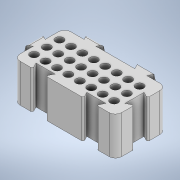
# Autodesk Inventor part: 4x11mmFlatBottom
Saved by Autodesk Inventor 2022.2 (Build 262287010, 287A)
## iProperties
Part Number: 4x11mmFlatBottom
Material: Generic
Document SubType Name: Modeling
Designer: yiunf
Appearance: Default
Author: yiunf
## iProperties of the stored document 4x8mm_3DPrint.ipt
Part Number: 4x8mm_3DPrint
Material: Generic
Document SubType Name: Modeling
Designer: yiunf
Appearance: Default
Author: yiunf
Autodesk Inventor part; units mm, degrees
ref_plane "YZ Plane" through (0, 0, 0) normal (1, 0, 0) x (0, 1, 0)
ref_plane "XZ Plane" through (0, 0, 0) normal (0, 1, 0) x (-1, 0, 0)
ref_plane "XY Plane" through (0, 0, 0) normal (0, 0, 1) x (1, 0, 0)
sketch "Sketch1" plane through (0, 0, 0) normal (0, 1, 0) x (-1, 0, 0)
  line L0 (-40, -20) -> (40, -20)
  line L1 (40, -20) -> (40, 20)
  line L2 (40, 20) -> (-40, 20)
  line L3 (-40, 20) -> (-40, -20)
  line L4 (-40, -20) -> (40, 20) construction
  line L5 (40, -20) -> (-40, 20) construction
  line L6 (40, 0) -> (45, 0)
  line L7 (45, 0) -> (45, 7.5)
  line L8 (40, 0) -> (40, 5)
  line L9 (40, 5) -> (45, 7.5)
  line L10 (45, 0) -> (45, -7.5)
  line L11 (40, 0) -> (40, -5)
  line L12 (40, -5) -> (45, -7.5)
  line L13 (0, -20) -> (5, -20)
  line L14 (0, -20) -> (-5, -20)
  line L15 (0, -20) -> (0, -25)
  line L16 (0, -25) -> (7.5, -25)
  line L17 (7.5, -25) -> (5, -20)
  line L18 (0, -25) -> (-7.5, -25)
  line L19 (-7.5, -25) -> (-5, -20)
  line L20 (-35, 0) -> (-35, -7.5)
  line L21 (-40, -5) -> (-35, -7.5)
  line L22 (-40, 0) -> (-35, 0)
  line L23 (-35, 0) -> (-35, 7.5)
  line L24 (-40, 5) -> (-35, 7.5)
  line L25 (-7.5, 15) -> (-5, 20)
  line L26 (0, 15) -> (-7.5, 15)
  line L27 (0, 20) -> (0, 15)
  line L28 (7.5, 15) -> (5, 20)
  line L29 (0, 15) -> (7.5, 15)
  line L30 (27.5, -25) -> (25, -20)
  line L31 (20, -25) -> (27.5, -25)
  line L32 (20, -25) -> (12.5, -25)
  line L33 (12.5, -25) -> (15, -20)
  line L34 (20, -20) -> (20, -25)
  line L35 (7.5, 15) -> (5, 20)
  line L36 (0, 15) -> (7.5, 15)
  line L37 (0, 15) -> (-7.5, 15)
  line L38 (-7.5, 15) -> (-5, 20)
  line L39 (0, 20) -> (0, 15)
  line L40 (27.5, 15) -> (25, 20)
  line L41 (20, 15) -> (27.5, 15)
  line L42 (20, 15) -> (12.5, 15)
  line L43 (12.5, 15) -> (15, 20)
  line L44 (20, 20) -> (20, 15)
  line L45 (-12.5, -25) -> (-15, -20)
  line L46 (-20, -25) -> (-12.5, -25)
  line L47 (-20, -20) -> (-20, -25)
  line L48 (-20, -25) -> (-27.5, -25)
  line L49 (-27.5, -25) -> (-25, -20)
  line L50 (7.5, 15) -> (5, 20)
  line L51 (0, 15) -> (7.5, 15)
  line L52 (0, 20) -> (0, 15)
  line L53 (0, 15) -> (-7.5, 15)
  line L54 (-7.5, 15) -> (-5, 20)
  line L55 (-12.5, 15) -> (-15, 20)
  line L56 (-20, 15) -> (-12.5, 15)
  line L57 (-20, 20) -> (-20, 15)
  line L58 (-20, 15) -> (-27.5, 15)
  line L59 (-27.5, 15) -> (-25, 20)
  line L60 (20, -24.75) -> (27.0955, -24.75)
  line L61 (27.0955, -24.75) -> (24.7764, -20.1118)
  line L62 (20, -24.75) -> (12.9045, -24.75)
  line L63 (12.9045, -24.75) -> (15.2236, -20.1118)
  line L64 (0, -24.5) -> (-6.691, -24.5)
  line L65 (-6.691, -24.5) -> (-4.691, -20.5)
  line L66 (-4.691, -20.5) -> (0, -20.5)
  line L67 (0, -24.75) -> (7.0955, -24.75)
  line L68 (7.0955, -24.75) -> (4.8455, -20.25)
  line L69 (4.8455, -20.25) -> (0, -20.25)
  line L70 (-20, -24.75) -> (-12.9045, -24.75)
  line L71 (-12.9045, -24.75) -> (-15.2236, -20.1118)
  line L72 (-20, -24.75) -> (-27.0955, -24.75)
  line L73 (-27.0955, -24.75) -> (-24.7764, -20.1118)
  line L74 (44.75, 0) -> (44.75, -7.0955)
  line L75 (44.75, -7.0955) -> (40.25, -4.8455)
  line L76 (40.25, -4.8455) -> (40.25, 0)
  line L77 (44.75, 0) -> (44.75, 7.0955)
  line L78 (44.75, 7.0955) -> (40.25, 4.8455)
  line L79 (40.25, 4.8455) -> (40.25, 0)
  line L80 (44.75, -7.0955) -> (40, -4.7205)
  line L81 (27.0955, -24.75) -> (24.7205, -20)
  line L82 (12.9045, -24.75) -> (15.2795, -20)
  line L83 (-12.9045, -24.75) -> (-15.2795, -20)
  line L84 (-27.0955, -24.75) -> (-24.7205, -20)
  line L85 (44.75, 7.0955) -> (40, 4.7205)
  line L86 (45, 0) -> (43.75, 0)
  line L87 (43.75, 0) -> (43.75, -6.875)
  line L88 (43.75, 0) -> (43.75, 6.875)
  line L89 (20, -25) -> (20, -23.75)
  line L90 (20, -23.75) -> (26.875, -23.75)
  line L91 (20, -23.75) -> (13.125, -23.75)
  line L92 (-20, -25) -> (-20, -23.75)
  line L93 (-20, -23.75) -> (-13.125, -23.75)
  line L94 (-20, -23.75) -> (-26.875, -23.75)
  point P0 (0, 0)
  point P1 (-40, -5)
  point P2 (24.7764, -20.1118)
  point P3 (40, -4.7205)
  point P4 (43.75, -6.5955)
  point P5 (43.75, 6.5955)
  point P6 (-26.5955, -23.75)
  point P7 (-13.4045, -23.75)
  point P8 (13.4045, -23.75)
  point P9 (26.5955, -23.75)
  dimension "d0" = 80
  dimension "d1" = 40
  dimension "d2" = 5
  dimension "d3" = 7.5
  dimension "d4" = 5
  dimension "d5" = 7.5
  dimension "d6" = 5
  dimension "d7" = 5
  dimension "d8" = 5
  dimension "d9" = 5
  dimension "d10" = 7.5
  dimension "d11" = 7.5
  dimension "d14" = 80
  dimension "d21" = 40
  dimension "d56" = 20
  dimension "d59" = 40
  dimension "d64" = 20
  dimension "d67" = 40
  dimension "d84" = 0.25
  dimension "d85" = 0.25
  dimension "d86" = 0.5
  dimension "d87" = 0.25
  dimension "d88" = 0.25
  dimension "d89" = 0.25
  dimension "d90" = 0.25
  dimension "d91" = 0.25
  dimension "d104" = 1.25
  dimension "d105" = 1.25
  dimension "d106" = 1.25
  constraints: 188 end point, 29 point on line, 12 horizontal alignment, 7 parallel, 6 vertical, 5 perpendicular, 4 collinear, 3 horizontal, 3 midpoint, 88 other
  measures "d0" distance of L2.end L1.end
  measures "d1" distance of L1.end L1.start
  measures "d2" distance of L6.start L6.end
  measures "d3" distance of L6.end L7.end
  measures "d4" distance of L6.start L8.end
  measures "d5" distance of L6.end L10.end
  measures "d6" distance of L6.start L11.end
  measures "d7" distance of L13.start L13.end
  measures "d8" distance of L13.start L14.end
  measures "d9" distance of L13.start L15.end
  measures "d10" distance of L15.end L16.end
  measures "d11" distance of L15.end L18.end
  measures "d14" distance of L10.end L20.end
  measures "d21" distance of L18.end L25.start
  measures "d56" distance of L16.end L30.start
  measures "d59" distance of L16.end L35.start
  measures "d64" distance of L16.end L45.start
  measures "d67" distance of L16.end L50.start
  measures "d84" distance between parallel lines of L31 L60
  measures "d85" distance between parallel lines of L32 L62
  measures "d86" distance between parallel lines of L18 L64
  measures "d87" distance between parallel lines of L16 L67
  measures "d88" distance between parallel lines of L46 L70
  measures "d89" distance between parallel lines of L48 L72
  measures "d90" distance between parallel lines of L10 L74
  measures "d91" distance between parallel lines of L7 L77
  measures "d104" distance of L6.end L86.end
  measures "d105" distance of L31.start L89.end
  measures "d106" distance of L46.start L92.end
extrude "Extrusion1" add sketch "Sketch1" along normal blind 30 contours L3 L21 L20 L23 L24 L2 L59 L58 L56 L55 L25 L26 L29 L28 L43 L42 L41 L40 L1 L0 | L0 L47 L94 L73 L84 | L0 L83 L71 L93 L47 | L2 L27 L26 L25 | L2 L28 L29 L27 | L0 L34 L91 L63 L82 | L0 L81 L61 L90 L34 | L1 L6 L76 L80 | L85 L79 L6 L1 | L76 L6 L87 L75 | L78 L88 L6 L79
sketch "Sketch2" plane through (0, 30, 0) normal (0, 1, 0) x (1, 0, 0)
  line L0 (-24.7205, 20) -> (-40, 20) projected
  line L1 (-40, 20) -> (-40, 10)
  line L2 (-40, 20) -> (-40, -20) projected
  line L3 (-40, 10) -> (-34, 10)
  circle A0 centre (-34, 10) radius 3.125
  circle A1 centre (-34, 0) radius 3.125
  circle A2 centre (-34, -10) radius 3.125
  circle A3 centre (-25, 10) radius 3.125
  circle A4 centre (-25, 0) radius 3.125
  circle A5 centre (-25, -10) radius 3.125
  circle A6 centre (-16, 10) radius 3.125
  circle A7 centre (-16, 0) radius 3.125
  circle A8 centre (-16, -10) radius 3.125
  circle A9 centre (-7, 10) radius 3.125
  circle A10 centre (-7, 0) radius 3.125
  circle A11 centre (-7, -10) radius 3.125
  circle A12 centre (2, 10) radius 3.125
  circle A13 centre (2, 0) radius 3.125
  circle A14 centre (2, -10) radius 3.125
  circle A15 centre (11, 10) radius 3.125
  circle A16 centre (11, 0) radius 3.125
  circle A17 centre (11, -10) radius 3.125
  circle A18 centre (20, 10) radius 3.125
  circle A19 centre (20, 0) radius 3.125
  circle A20 centre (20, -10) radius 3.125
  circle A21 centre (29, 10) radius 3.125
  circle A22 centre (29, 0) radius 3.125
  circle A23 centre (29, -10) radius 3.125
  point P0 (-40, 4.7205)
  dimension "d92" = 10
  dimension "d93" = 6
  dimension "d95" = 6.25
  dimension "d98" = 10
  dimension "d101" = 9
  constraints: 24 centre point, 4 end point, 1 coincident, 1 horizontal, 1 perpendicular, 1 point on line, 1 vertical, 46 other
  measures "d92" distance of L0.end L1.end
  measures "d93" distance of L1.end L3.end
  measures "d95" diameter of A0
  measures "d98" distance of A0.centre A1.centre
  measures "d101" distance of A0.centre A3.centre
extrude "Extrusion2" cut sketch "Sketch2" against normal blind 20
fillet "Fillet1" radius 1 6 edges at (40, 15, -5) (40, 15, 5) (25, 15, 20) (15, 15, 20) (-15, 15, 20) (-25, 15, 20)
fillet "Fillet2" radius 5 4 edges at (40, 15, -20) (40, 15, 20) (-40, 15, 20) (-40, 15, -20)
ref_plane "Work Plane1" through (-43.75, 0, 6.5955) normal (0, 0, 1) x (0, 1, 0)
sketch "Sketch3" plane through (-43.75, 0, 6.5955) normal (0, 0, 1) x (0, 1, 0)
  line L0 (0, -3.75) -> (30, -3.75) projected
  line L1 (15, -3.75) -> (15, 2)
  line L2 (0, 0) -> (30, 0) projected
  arc A0 (30, 0) -> (0, 0) centre (15, -55.25) ccw
  line L3 (30, 0) -> (30, -3.75) projected
  line L4 (30, 0) -> (25, 0)
  line L5 (25, 0) -> (5, 0)
  line L6 (15, 2) -> (15, 1)
  arc A1 (25, 0) -> (5, 0) centre (15, -49.5) ccw
  point P0 (0, -43.75)
  dimension "d108" = 5.75
  dimension "d109" = 5
  dimension "d110" = 20
  dimension "d111" = 1
  constraints: 8 end point, 6 point on circle, 3 point on line, 2 centre point, 1 midpoint, 1 vertical
  measures "d108" distance of L1.start L1.end
  measures "d109" distance of L2.end L4.end
  measures "d110" distance of L4.end L5.end
  measures "d111" distance of L1.end L6.end
extrude "Extrusion3" add sketch "Sketch3" against normal blind 13.191 contours L2 A1 L1 A0 | A1 L2 A0 L1
sketch "Sketch4" plane through (0, 30, 0) normal (0, 1, 0) x (1, 0, 0)
  line L0 (-13.4045, 23.75) -> (-26.5955, 23.75) projected
  line L1 (-20, 23.75) -> (-20, -15)
  line L2 (-27.5, -15) -> (-12.5, -15) projected
  line L3 (-43.75, 6.5955) -> (-43.75, -6.5955) projected
  line L4 (-43.75, 0) -> (-20, 0)
  line L5 (13.4045, 23.75) -> (15.2795, 20) projected
  line L6 (-43.75, -6.5955) -> (-40, -4.7205) projected
  line L7 (26.5955, 23.75) -> (13.4045, 23.75) projected
  line L8 (-40, 4.7205) -> (-43.75, 6.5955) projected
  line L9 (24.7205, 20) -> (26.5955, 23.75) projected
  point P0 (0, 0)
  point P1 (-43.75, 6.5955)
  constraints: 4 end point, 3 midpoint, 1 perpendicular, 1 point on line
fillet "Fillet3" radius 2 2 edges at (-43.75, 30, 0) (-43.75, 0, 0)
pattern_circular "Circular Pattern1" count 2 over 270 about axis through (-20, 30, 0) along (0, 1, 0) of "Fillet3", "Extrusion3"
ref_plane "Work Plane3" through (26.5955, 0, -23.75) normal (-1, 0, 0) x (0, 1, 0)
sketch "Sketch6" plane through (26.5955, 0, -23.75) normal (-1, 0, 0) x (0, 1, 0)
  line L0 (0, -3.75) -> (30, -3.75) projected
  line L1 (15, -3.75) -> (15, 2)
  line L2 (0, 0) -> (30, 0) projected
  arc A0 (30, 0) -> (0, 0) centre (15, -55.25) ccw
  arc A1 (25, 0) -> (5, 0) centre (15, -49.5) ccw projected
  arc A2 (25, 0) -> (5, 0) centre (15, -49.5) ccw
  point P0 (0, -23.75)
  dimension "d120" = 5.75
  constraints: 5 point on circle, 2 centre point, 2 end point, 1 midpoint, 1 vertical
  measures "d120" distance of L1.start L1.end
extrude "Extrusion4" add sketch "Sketch6" along normal blind 13.191 contours A1 L2 A0 L1 | L1 A0 L2 A1
body "Solid1"
